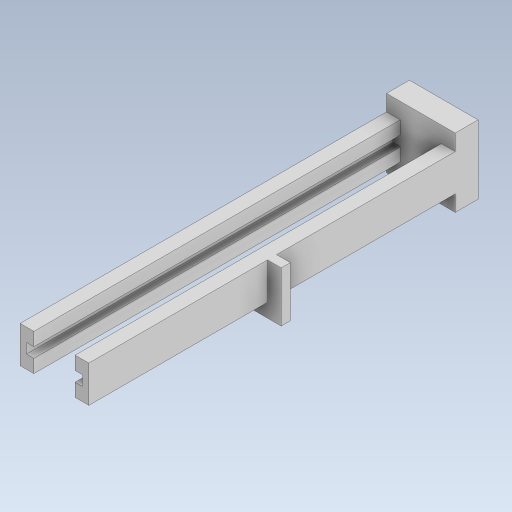
# Autodesk Inventor part: Bracket Lifter
Saved by Autodesk Inventor 2023.5 (Build 275446000, 446)
## iProperties
Created: 2025-09-02
Part Number: Bracket Lifter
Material: Generic
Document SubType Name: Modeling
Designer: Guntur
Density: 1 g/cm^3
Appearance: Default
Author: Guntur
Autodesk Inventor part; units mm, degrees
ref_plane "YZ Plane" through (0, 0, 0) normal (1, 0, 0) x (0, 1, 0)
ref_plane "XZ Plane" through (0, 0, 0) normal (0, 1, 0) x (-1, 0, 0)
ref_plane "XY Plane" through (0, 0, 0) normal (0, 0, 1) x (1, 0, 0)
sketch "Sketch1" plane through (0, 0, 0) normal (0, 0, 1) x (1, 0, 0)
  line L0 (-7.5, 7.5) -> (7.5, 7.5)
  line L1 (7.5, 7.5) -> (7.5, -7.5)
  line L2 (7.5, -7.5) -> (-7.5, -7.5)
  line L3 (-7.5, -7.5) -> (-7.5, 7.5)
  line L4 (-7.5, 7.5) -> (7.5, -7.5) construction
  line L5 (7.5, 7.5) -> (-7.5, -7.5) construction
  line L6 (0, 4.0776) -> (0, -3.6051) construction
  line L7 (-7.5, 4) -> (-4.5, 4)
  line L8 (-4.5, -4) -> (-7.5, -4)
  line L9 (-7.5, -4) -> (-7.5, 4)
  line L10 (-7.5, 4) -> (-4.5, -4) construction
  line L11 (-4.5, 4) -> (-7.5, -4) construction
  line L12 (-6.1, 1.1) -> (-4.5, 1.1)
  line L13 (-2.9, 1.1) -> (-2.9, -1.1)
  line L14 (-4.5, -1.1) -> (-6.1, -1.1)
  line L15 (-6.1, -1.1) -> (-6.1, 1.1)
  line L16 (-6.1, 1.1) -> (-2.9, -1.1) construction
  line L17 (-2.9, 1.1) -> (-6.1, -1.1) construction
  line L18 (7.5, 7.5) -> (-7.5, -7.5) construction
  line L19 (-7.5, 7.5) -> (7.5, -7.5) construction
  line L20 (7.5, 4) -> (4.5, 4)
  line L21 (4.5, -4) -> (7.5, -4)
  line L22 (7.5, 4) -> (4.5, -4) construction
  line L23 (4.5, 4) -> (7.5, -4) construction
  line L24 (6.1, 1.1) -> (4.5, 1.1)
  line L25 (4.5, -1.1) -> (6.1, -1.1)
  line L26 (6.1, -1.1) -> (6.1, 1.1)
  line L27 (6.1, 1.1) -> (2.9, -1.1) construction
  line L28 (2.9, 1.1) -> (6.1, -1.1) construction
  line L29 (4.5, 4) -> (4.5, 1.1)
  line L30 (4.5, -1.1) -> (4.5, -4)
  line L31 (-4.5, 4) -> (-4.5, 1.1)
  line L32 (-4.5, -1.1) -> (-4.5, -4)
  point P0 (0, 0)
  point P1 (-6, 0)
  point P2 (-4.5, 0)
  point P3 (6, 0)
  point P4 (4.5, 0)
  dimension "d0" = 15
  dimension "d1" = 15
  dimension "d2" = 3
  dimension "d3" = 8
  dimension "d6" = 3.2
  dimension "d7" = 2.2
  constraints: 66 end point, 14 symmetric about line, 8 midpoint, 7 parallel, 4 perpendicular, 3 horizontal, 2 vertical
  measures "d0" distance of L1.end L2.end
  measures "d1" distance of L0.end L1.end
  measures "d2" distance of L8.start L8.end
  measures "d3" distance of L7.end L8.start
  measures "d6" distance of L13.end L14.end
  measures "d7" distance of L13.start L13.end
extrude "Extrusion1" add sketch "Sketch1" against normal blind 5
extrude "Extrusion2" add sketch "Sketch1" along normal blind 80 contours L7 L31 L12 L15 L14 L32 L8 L3 | L1 L21 L30 L25 L26 L24 L29 L20
sketch "Sketch2" plane through (4.5, -4, 0) normal (0, -1, 0) x (1, 0, 0)
  line L0 (3, 0) -> (3, 80) projected
  line L1 (-3, 41) -> (3, 41)
  line L2 (3, 41) -> (3, 39)
  line L3 (3, 39) -> (-3, 39)
  line L4 (-3, 39) -> (-3, 41)
  line L5 (0, 0) -> (0, 80) projected
  line L6 (-3, 41) -> (3, 39) construction
  line L7 (3, 41) -> (-3, 39) construction
  line L8 (0, 41) -> (0, 39)
  point P0 (-4.5, 0)
  point P1 (0, 40)
  point P2 (3, 41)
  dimension "d12" = 2
  constraints: 14 end point, 5 midpoint, 3 point on line, 2 parallel, 1 horizontal, 1 perpendicular
  measures "d12" distance of L1.end L2.end
extrude "Extrusion3" add sketch "Sketch2" along normal blind 3 contours L3 L5 L1 L0
sketch "Sketch3" plane through (7.5, -7.5, -5) normal (1, 0, 0) x (0, 0, -1)
  line L0 (-44, 0.5) -> (-46, 0.5) projected
  line L1 (-5, 11.5) -> (-85, 11.5) projected
  line L2 (-46, 0.5) -> (-44, 0.5)
  line L3 (-44, 0.5) -> (-44, 11.5)
  line L4 (-44, 11.5) -> (-46, 11.5)
  line L5 (-46, 11.5) -> (-46, 0.5)
  point P0 (-5, 7.5)
  dimension "d15" = 2
  constraints: 8 end point, 2 parallel, 1 horizontal, 1 perpendicular, 1 point on line
  measures "d15" distance of L4.end L3.end
extrude "Extrusion4" add sketch "Sketch3" along normal blind 3
body "Solid1"
